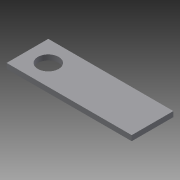
# Autodesk Inventor part: BarHolder
Saved by Autodesk Inventor 2013 (Build 170138000, 138)
## iProperties
Created: 2014-01-18
Part Number: BarHolder
Material: Generic
Document SubType Name: Modeling
Designer: 272817
Density: 1 g/cm^3
Author: 272817
Autodesk Inventor part; units mm, degrees
ref_plane "YZ Plane" through (0, 0, 0) normal (1, 0, 0) x (0, 1, 0)
ref_plane "XZ Plane" through (0, 0, 0) normal (0, 1, 0) x (-1, 0, 0)
ref_plane "XY Plane" through (0, 0, 0) normal (0, 0, 1) x (1, 0, 0)
sketch "Sketch1" plane through (0, 0, 0) normal (0, 1, 0) x (-1, 0, 0)
  line L0 (-76.2, -12.7) -> (76.2, -12.7)
  line L1 (76.2, -12.7) -> (76.2, 12.7)
  line L2 (76.2, 12.7) -> (-76.2, 12.7)
  line L3 (-76.2, 12.7) -> (-76.2, -12.7)
  line L4 (-76.2, -12.7) -> (76.2, 12.7) construction
  line L5 (76.2, -12.7) -> (-76.2, 12.7) construction
  line L6 (-76.2, 0) -> (-63.5, 0)
  line L7 (-76.2, 0) -> (-63.5, 0) construction
  line L8 (76.2, 0) -> (50.8, 0)
  line L9 (76.2, 0) -> (101.6, 0) construction
  line L10 (50.8, 0) -> (25.4, 0)
  circle A0 centre (-63.5, 0) radius 3.175
  circle A1 centre (25.4, 0) radius 3.175
  point P0 (0, 0)
  dimension "d0" = 152.4
  dimension "d1" = 25.4
  dimension "d2" = 12.7
  dimension "d3" = 0
  dimension "d4" = 25.4
  dimension "d5" = 180
  dimension "d6" = 25.4
  dimension "d7" = 6.35
  dimension "d8" = 6.35
  constraints: 22 end point, 4 coincident, 4 collinear, 4 midpoint, 3 horizontal, 2 centre point, 2 parallel, 2 perpendicular
  measures "d0" distance of L2.end L1.end
  measures "d1" distance of L1.end L0.end
  measures "d2" distance of L6.start L6.end
  measures "d3" distance between parallel lines of L6 L7
  measures "d4" distance of L8.start L8.end
  measures "d5" angle of L8 L9
  measures "d6" distance of L8.end L10.end
  measures "d7" diameter of A0
  measures "d8" diameter of A1
extrude "Extrusion1" add sketch "Sketch1" along normal blind 3.175
sketch "Sketch2" plane through (0, 3.175, 0) normal (0, 1, 0) x (1, 0, 0)
  circle A0 centre (-63.5, 0) radius 3.175
  point P0 (0, 0)
  dimension "d11" = 6.35
  constraints: 1 centre point
  measures "d11" diameter of A0
extrude "Extrusion2" cut sketch "Sketch2" against normal blind 25.4
sketch "Sketch3" plane through (0, 3.175, 0) normal (0, 1, 0) x (1, 0, 0)
  circle A0 centre (-63.5, 0) radius 3.175 projected
  circle A1 centre (-63.5, 0) radius 6.35
  point P0 (0, 0)
  dimension "d14" = 12.7
  constraints: 1 centre point, 1 coincident
  measures "d14" diameter of A1
extrude "Extrusion3" cut sketch "Sketch3" against normal blind 25.4
sketch "Sketch4" plane through (0, 3.175, 0) normal (0, 1, 0) x (1, 0, 0)
  circle A0 centre (63.5, 0) radius 3.175 projected
  line L0 (76.2, 12.7) -> (-76.2, 12.7) projected
  line L1 (-76.2, -12.7) -> (76.2, -12.7) projected
  line L2 (76.2, -12.7) -> (76.2, 12.7) projected
  line L3 (0, 12.7) -> (0, -12.7)
  point P0 (0, 0)
  constraints: 2 end point, 2 midpoint
extrude "Extrusion4" cut sketch "Sketch4" against normal blind 25.4
sketch "Sketch5" plane through (0, 3.175, 0) normal (0, 1, 0) x (1, 0, 0)
  circle A0 centre (-25.4, 0) radius 3.175 projected
  circle A1 centre (-25.4, 0) radius 3.175
  point P0 (0, 0)
  constraints: 1 centre point, 1 coincident, 1 concentric
extrude "Extrusion5" add sketch "Sketch5" against normal blind 3.175
body "Solid1"
